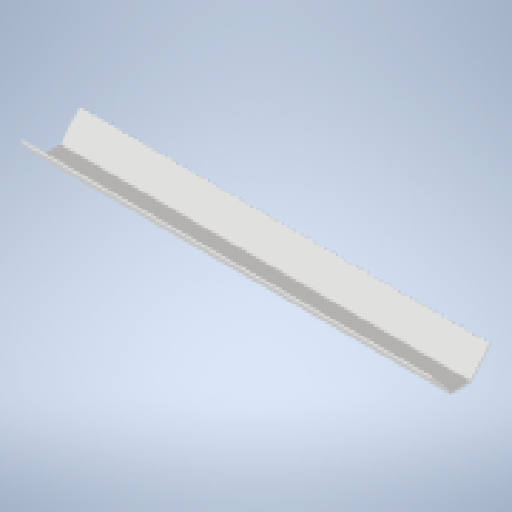
# Autodesk Inventor part: DF 4.1 Tray
Saved by Autodesk Inventor 2024.2 (Build 282272000, 272)
## iProperties
Created: 2023-09-04
Part Number: DF 4.1 Tray
Material: Generic
Document SubType Name: Sheet Metal
Designer: admin
Density: 1 g/cm^3
Sheet Metal Rule: Default_mm
Appearance: Default
Author: admin
Autodesk Inventor part; units mm, degrees
ref_plane "YZ Plane" through (0, 0, 0) normal (1, 0, 0) x (0, 1, 0)
ref_plane "XZ Plane" through (0, 0, 0) normal (0, 1, 0) x (-1, 0, 0)
ref_plane "XY Plane" through (0, 0, 0) normal (0, 0, 1) x (1, 0, 0)
sketch "Sketch1" plane through (0, 0, 0) normal (0, 1, 0) x (-1, 0, 0)
  line L0 (-990, -50) -> (990, -50)
  line L1 (990, -50) -> (990, 50)
  line L2 (990, 50) -> (-990, 50)
  line L3 (-990, 50) -> (-990, -50)
  line L4 (-990, -50) -> (990, 50) construction
  line L5 (990, -50) -> (-990, 50) construction
  point P0 (0, 0)
  dimension "d0" = 1980
  dimension "d1" = 100
  constraints: 12 end point, 2 midpoint, 2 parallel, 1 horizontal, 1 perpendicular
  measures "d0" distance of L1.end L2.end
  measures "d1" distance of L2.end L0.start
extrude "Plate1" add sketch "Sketch1" along normal blind 10
sketch "Sketch2" plane through (990, 6.4279, 42.3396) normal (0, -0.6427876, 0.7660444) x (1, 0, 0)
  line L0 (-1980, 0) -> (0, 0)
  line L1 (0, 0) -> (0, 150)
  line L2 (0, 150) -> (-1980, 150)
  line L3 (-1980, 150) -> (-1980, 0)
  constraints: 6 end point, 1 horizontal, 1 perpendicular, 1 vertical
edge flange "Flange1" height 150 angle 50 thickness 10 bend radius 10 thickness toward (0, -0.6427876, 0.7660444) relief straight relief width 10 relief depth 5 corner gap 10 corner form 0 edges at (0, 10, 50) (0, 10, -50) wall of the first edge with corners at (-990, 6.4279, 42.3396) (990, 6.4279, 42.3396) (990, 121.3345, 138.7577) (-990, 121.3345, 138.7577)
bend "Bend1"
corner "Corner1"
equation "\"d2\" = Thickness"
equation "\"d3\" = BendReliefWidth"
equation "\"d4\" = BendReliefDepth"
equation "\"d5\" = MinimumRemnant"
equation "\"d6\" = TransitionRadius"
equation "\"d9\" = BendRadius"
equation "\"d10\" = CornerReliefSize"
equation "\"d11\" = GapSize"
equation "\"d12\" = JacobiRadiusSize"
equation "\"BendRadius\" = Thickness"
equation "\"BendReliefDepth\" = 0.5 * Thickness"
equation "\"Thickness\" = 10"
equation "\"BendReliefWidth\" = 10"
equation "\"MinimumRemnant\" = 20"
equation "\"TransitionRadius\" = 10"
equation "\"CornerReliefSize\" = 40"
equation "\"GapSize\" = 10"
equation "\"JacobiRadiusSize\" = 10"
body "Solid1"
